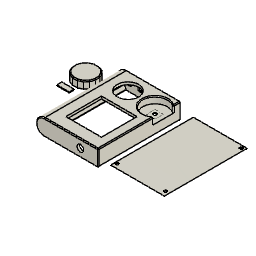
Luxer_main v10 (Autodesk Fusion 360 design; units mm, degrees)
Autodesk Fusion 360 part; units mm, degrees
sketch "草图1" plane through (0, 0, 0) normal (0, 0, 1) x (1, 0, 0)
  line L0 (-40.0171, 49.9772) -> (34.9829, 49.9772)
  line L1 (34.9829, 49.9772) -> (34.9829, -50.0228)
  line L2 (34.9829, -50.0228) -> (-40.0171, -50.0228)
  line L3 (-40.0171, -50.0228) -> (-40.0171, 49.9772)
  circle A0 centre (-8, 29) radius 13
  line L4 (-18.3671, 7.3548) -> (24.6329, 7.3548)
  line L5 (24.6329, 7.3548) -> (24.6329, -35.6452)
  line L6 (24.6329, -35.6452) -> (-18.3671, -35.6452)
  line L7 (-18.3671, -35.6452) -> (-18.3671, 7.3548)
  line L8 (33.5, 48.5) -> (-30, 48.5)
  line L9 (-30, 48.5) -> (-30, -47)
  line L10 (-30, -47) -> (33.5, -47)
  arc A1 (34.9829, 39.8827) -> (34.9829, 18.1173) centre (24.6597, 29) ccw
  arc A2 (34.9829, 41.8647) -> (34.9829, 16.1353) centre (24.6597, 29) ccw
  line L11 (33.5, -47) -> (33.5, 15.0746)
  line L12 (33.5, 42.9254) -> (33.5, 48.5)
  line L13 (33.5, 42.9254) -> (33.5, 15.0746)
  circle A3 centre (24.6597, 29) radius 2
  line L14 (29.7597, 23.9) -> (19.5597, 23.9)
  line L15 (19.5597, 23.9) -> (19.5597, 34.1)
  line L16 (19.5597, 34.1) -> (29.7597, 34.1)
  line L17 (29.7597, 34.1) -> (29.7597, 23.9)
  line L18 (29.7597, 23.9) -> (19.5597, 34.1) construction
  line L19 (19.5597, 23.9) -> (29.7597, 34.1) construction
  circle A4 centre (31.5, 46.5) radius 1.85
  arc A5 (29.5, 48.5) -> (29.4957, 44.7696) centre (30.7332, 46.6334) ccw
  circle A6 centre (30.6894, -44.1882) radius 1.85
  circle A7 centre (-27.5, -44.5) radius 1.85
  arc A8 (-23.5, -47) -> (-30, -40.5) centre (-30, -47) ccw
  arc A9 (33.5, -40) -> (26.5, -47) centre (33.5, -47) ccw
  line L20 (-30, -47) -> (-30, -50.0228)
  line L21 (-30, 48.5) -> (-30, 49.9772)
  point P0 (24.6597, 29)
  dimension "d2" = 75
  dimension "d3" = 100
  dimension "d4" = 26
  dimension "d5" = 15
  dimension "d6" = 43
  dimension "d7" = 43
  dimension "d32" = 4
  dimension "d33" = 10.2
  dimension "d34" = 10.2
  dimension "d63" = 3.7
  dimension "d65" = 3.7
  dimension "d66" = 3.7
  constraint horizontal L0
  constraint vertical L1
  constraint horizontal L2
  constraint vertical L3
  constraint horizontal L4
  constraint vertical L5
  constraint horizontal L6
  constraint vertical L7
  constraint horizontal A0.centre P0
  constraint horizontal L8
  constraint vertical L9
  constraint horizontal L10
  constraint vertical L11
  constraint concentric A1 A2
  constraint coincident L1 A1.end
  constraint coincident L1 A1.start
  constraint coincident L1 A2.end
  constraint coincident L1 A2.start
  constraint coincident A2 L12.start
  constraint collinear L11 L12
  constraint coincident A2 L11.end
  constraint concentric A2 A3
  constraint perpendicular L14 L15
  constraint parallel L14 L16
  constraint parallel L15 L17
  constraint horizontal L14
  constraint coincident L18 P0
  constraint coincident L19 P0
  constraint coincident P0 A1.centre
  constraint coincident L8 A5.start
  constraint coincident A2 A5.end
  constraint coincident L10 A8.start
  constraint coincident L9.end L10.start
  constraint coincident L9 A8.end
  constraint coincident L10 A9.end
  constraint coincident L10.end L11.start
  constraint coincident L11 A9.start
  constraint coincident L2 L20.end
  constraint perpendicular L2 L20
  constraint coincident L0 L21.end
  constraint perpendicular L0 L21
  measures "d2" distance of L0.start L0.end
  measures "d3" distance of L0.start L2.end
  measures "d4" diameter of A0
  measures "d5" radius of A1
  measures "d6" distance of L4.start L4.end
  measures "d7" distance of L4.start L6.end
  measures "d32" diameter of A3
  measures "d33" distance of L15.end L16.end
  measures "d34" distance of L14.end L15.end
  measures "d63" diameter of A4
  measures "d65" diameter of A6
  measures "d66" diameter of A7
extrude "拉伸4" add sketch "草图1" along normal mid plane 20 contours L0 L2 L3 L9 L20 L21 | L0 L1 L8 A2 L12 L21 | L8 L9 L10 A2 L11 A5 A8 A9 | L1 L2 L10 A2 L11 L20 | L1 A1 A2 L13 | L8 A2 L12 A5 | L9 L10 A8 | L1 A1 L13 | A1 A2 L13 | L1 A1 A2 L13 | A1 L13 | L10 L11 A9 | A0 | L4 L5 L6 L7 | A3 | L14 L15 L16 L17 | A4 | A6 | A7 makes body 1
extrude "拉伸5" cut sketch "草图1" along normal blind 17 from surface at -10 contours L8 L9 L10 A2 L11 A5 A8 A9 | L8 A2 L12 A5 | L9 L10 A8 | L10 L11 A9 | A4 | A6 | A7 bodies 1
extrude "拉伸6" add sketch "草图1" along normal blind 17 from surface at -10 contours L8 L9 L10 A2 L11 A5 A8 A9 | L8 A2 L12 A5 | L9 L10 A8 | L10 L11 A9 | A4 | A6 | A7 bodies 1
extrude "拉伸7" cut sketch "草图1" along normal blind 17 from surface at -10 contours L8 L9 L10 A2 L11 A5 A8 A9 | L8 A2 L12 A5 | L9 L10 A8 | L10 L11 A9 | A4 | A6 | A7 bodies 1
extrude "拉伸8" cut sketch "草图1" against normal blind 20 from surface at 10 contours L4 L5 L6 L7 bodies 1
extrude "拉伸9" cut sketch "草图1" against normal blind 20 from surface at 10 contours A0 bodies 1
extrude "拉伸10" cut sketch "草图1" against normal blind 8 from surface at 10 contours L1 A1 L13 | A1 L13 | A3 | L14 L15 L16 L17 bodies 1
extrude "拉伸11" cut sketch "草图1" along normal blind 8 from surface at -10 contours A1 A2 L13 | A1 L13 | A3 | L14 L15 L16 L17 bodies 1
extrude "拉伸12" cut sketch "草图1" along normal blind 3 from surface at -2 contours A3 | L14 L15 L16 L17 bodies 1
extrude "拉伸13" cut sketch "草图1" along normal blind 5 contours A3 bodies 1
fillet "圆角1" radius 10 1 edges at (-40.0171, -0.0228, 10) on bodies 1
fillet "圆角2" radius 10 1 edges at (-40.0171, -0.0228, -10) on bodies 1
fillet "圆角3" radius 1.5 1 edges at (34.9829, -0.0228, -10) on bodies 1
sketch "草图2" plane through (0, 0, 0) normal (0, 1, 0) x (1, 0, 0)
  circle A0 centre (13.5508, -0.0658) radius 4
  circle A1 centre (-26, 0) radius 3.75
  line L0 (4.004, -3.3409) -> (-15.196, -3.3409)
  line L1 (-15.196, -3.3409) -> (-15.196, 3.4591)
  line L2 (-15.196, 3.4591) -> (4.004, 3.4591)
  line L3 (4.004, 3.4591) -> (4.004, -3.3409)
  line L4 (4.004, -3.3409) -> (-15.196, 3.4591) construction
  line L5 (-15.196, -3.3409) -> (4.004, 3.4591) construction
  point P0 (-5.596, 0.0591)
  dimension "d50" = 8
  dimension "d51" = 7.5
  dimension "d84" = 19.2
  dimension "d85" = 6.8
  constraint perpendicular L0 L1
  constraint parallel L0 L2
  constraint parallel L1 L3
  constraint horizontal L0
  constraint coincident L4 P0
  constraint coincident L5 P0
  measures "d50" diameter of A0
  measures "d51" diameter of A1
  measures "d84" distance of L1.end L2.end
  measures "d85" distance of L0.end L1.end
extrude "拉伸23" add sketch "草图1" against normal blind 17 from surface at 7 contours L10 L11 A9 bodies 1
extrude "拉伸24" add sketch "草图1" against normal blind 17 from surface at 7 contours L9 L10 A8 bodies 1
extrude "拉伸25" add sketch "草图1" against normal blind 17 from surface at 7 contours L8 A2 L12 A5 bodies 1
extrude "拉伸26" cut sketch "草图2" along normal blind 58 contours L0 L1 L2 L3 bodies 1
extrude "拉伸27" cut sketch "草图2" along normal blind 57 contours A1 bodies 1
extrude "拉伸28" cut sketch "草图2" against normal blind 60 contours A0 bodies 1
extrude "拉伸29" add sketch "草图1" along normal mid plane 1.4 separate body contours L0 L1 L8 A2 L12 L21 | L8 L9 L10 A2 L11 A5 A8 A9 | L1 L2 L10 A2 L11 L20 | L1 A1 A2 L13 | L8 A2 L12 A5 | L9 L10 A8 | L1 A1 L13 | A1 A2 L13 | L1 A1 A2 L13 | A1 L13 | L10 L11 A9 | A0 | L4 L5 L6 L7 makes body 2
move_body "移动1" bodies 2 to x (1, 0, 0) y (0, 1, 0) z (0, 0, 1) at (80, 0, 0)
delete_face "删除面4" 1 faces at (106.3597, 34.1, -0.2333) on bodies 2
chamfer "倒角1" distance 0.3 angle 45 1 edges at (109.7752, 45.831, -0.7) on bodies 2
chamfer "倒角2" distance 0.3 angle 45 1 edges at (108.9646, -44.8572, -0.7) on bodies 2
chamfer "倒角3" distance 0.3 angle 45 1 edges at (50.7752, -45.169, -0.7) on bodies 2
sketch "草图3" plane through (0, 0, 0) normal (0, 0, 1) x (1, 0, 0)
  line L0 (-51.8552, 41.0396) -> (-57.0064, 42.8573)
  line L1 (-57.0064, 42.8573) -> (-62.4611, 42.5654)
  line L2 (-62.4611, 42.5654) -> (-67.3889, 40.2083)
  line L3 (-67.3889, 40.2083) -> (-71.0396, 36.1448)
  line L4 (-71.0396, 36.1448) -> (-72.8573, 30.9936)
  line L5 (-72.8573, 30.9936) -> (-72.5654, 25.5389)
  line L6 (-72.5654, 25.5389) -> (-70.2083, 20.6111)
  line L7 (-70.2083, 20.6111) -> (-66.1448, 16.9604)
  line L8 (-66.1448, 16.9604) -> (-60.9936, 15.1427)
  line L9 (-60.9936, 15.1427) -> (-55.5389, 15.4346)
  line L10 (-55.5389, 15.4346) -> (-50.6111, 17.7917)
  line L11 (-50.6111, 17.7917) -> (-46.9604, 21.8552)
  line L12 (-46.9604, 21.8552) -> (-45.1427, 27.0064)
  line L13 (-45.1427, 27.0064) -> (-45.4346, 32.4611)
  line L14 (-45.4346, 32.4611) -> (-47.7917, 37.3889)
  line L15 (-47.7917, 37.3889) -> (-51.8552, 41.0396)
  circle A0 centre (-59, 29) radius 1.95
  circle A1 centre (-59, 29) radius 11
  circle A2 centre (-59, 29) radius 5
  line L16 (-66.6051, 1.6351) -> (-51.6051, 1.6351)
  line L17 (-51.6051, 1.6351) -> (-51.6051, 7.6351)
  line L18 (-51.6051, 7.6351) -> (-66.6051, 7.6351)
  line L19 (-66.6051, 7.6351) -> (-66.6051, 1.6351)
  point P0 (-59, 29)
  dimension "d108" = 14
  dimension "d109" = 3.9
  dimension "d125" = 13.8573
  dimension "d126" = 15
  dimension "d127" = 6
  dimension "d128" = 10
  constraint coincident P0 A0.centre
  constraint horizontal L16
  constraint vertical L17
  constraint horizontal L18
  constraint vertical L19
  measures "d108" distance of L0.start P0
  measures "d109" diameter of A0
  measures "d125" horizontal distance of L4.end P0
  measures "d126" distance of L17.end L18.end
  measures "d127" distance of L16.start L18.end
  measures "d128" diameter of A2
extrude "拉伸30" add sketch "草图3" along normal mid plane 9 separate body contours L0 L1 L2 L3 L4 L5 L6 L7 L8 L9 L10 L11 L12 L13 L14 L15 | A0 | A1 | A2 makes body 3
extrude "拉伸31" cut sketch "草图3" along normal blind 7.5 from surface at -4.5 contours A0 bodies 3
extrude "拉伸32" cut sketch "草图3" along normal blind 7.5 from surface at -4.5 contours A1 bodies 3
chamfer "倒角4" distance 1 angle 45 16 edges at (-53.075, 16.6131, 4.5) (-48.7857, 19.8235, 4.5) (-46.0515, 24.4308, 4.5) (-45.2886, 29.7338, 4.5) (-46.6131, 34.925, 4.5) (-49.8235, 39.2143, 4.5) (-54.4308, 41.9485, 4.5) (-59.7338, 42.7114, 4.5) (-64.925, 41.3869, 4.5) (-69.2143, 38.1765, 4.5) (-71.9485, 33.5692, 4.5) (-72.7114, 28.2662, 4.5) (-71.3869, 23.075, 4.5) (-68.1765, 18.7857, 4.5) (-63.5692, 16.0515, 4.5) (-58.2662, 15.2886, 4.5) on bodies 3
fillet "圆角4" radius 0.5 16 edges at (-71.9485, 33.5692, -4.5) (-69.2143, 38.1765, -4.5) (-64.925, 41.3869, -4.5) (-59.7338, 42.7114, -4.5) (-54.4308, 41.9485, -4.5) (-72.7114, 28.2662, -4.5) (-71.3869, 23.075, -4.5) (-68.1765, 18.7857, -4.5) (-63.5692, 16.0515, -4.5) (-58.2662, 15.2886, -4.5) (-53.075, 16.6131, -4.5) (-48.7857, 19.8235, -4.5) (-46.0515, 24.4308, -4.5) (-45.2886, 29.7338, -4.5) (-46.6131, 34.925, -4.5) (-49.8235, 39.2143, -4.5) on bodies 3
extrude "拉伸33" cut 1 faces at (-55.0425, 28.6547, -4.5) along direction (0, 0, 1) blind 0.5 on bodies 3 bodies 3
fillet "圆角5" radius 1.5 4 edges at (114.9829, -0.0228, -0.7) (50, -0.0228, -0.7) (82.4914, -50.0228, -0.7) (82.4914, 49.9772, -0.7) on bodies 2
extrude "拉伸34" add sketch "草图3" along normal mid plane 1 separate body contours L16 L17 L18 L19 makes body 4
fillet "圆角6" radius 1 2 edges at (34.9829, 18.1173, 6) (34.9829, 39.8827, 6) on bodies 1
chamfer "倒角5" distance 1 angle 45 15 edges at (34.9829, -17.0129, 10) (34.4397, 16.8865, 10) (9.6597, 29, 10) (34.4397, 41.1135, 10) (34.9829, 45.9901, 10) (2.4829, 49.9772, 10) (-40.0171, 49.9772, 0) (1.7329, 49.9772, -10) (34.5435, 49.9772, -9.5607) (34.9829, 49.9772, 0.75) (34.9829, -50.0228, 0.75) (34.5435, -50.0228, -9.5607) (1.7329, -50.0228, -10) (-40.0171, -50.0228, 0) (2.4829, -50.0228, 10) on bodies 1
cylinder "圆柱体基本要素1" cut diameter 12.5 height 85 placed x (1, 0, 0) y (0, 0, 1) z (0, -1, 0) at (-30, 48.5, 0) bodies 1
fillet "圆角7" radius 1 2 edges at (-30, 6, 6.25) (-30, 4, 7) on bodies 1
fillet "圆角8" radius 4 1 edges at (-30, 6, -6.25) on bodies 1
delete_face "删除面5" 1 faces at (-22.2686, 49.4848, -0.3734) on bodies 1
extrude "拉伸35" cut sketch "草图2" along normal blind 73 contours A1 bodies 1
fillet "圆角9" radius 2 1 edges at (-29.9683, 6, 6.2499) on bodies 1
extrude "拉伸14" [suppressed]
extrude "拉伸15" [suppressed]
extrude "拉伸16" [suppressed]
extrude "拉伸17" [suppressed]
extrude "拉伸18" [suppressed]
extrude "拉伸19" [suppressed]
extrude "拉伸20" [suppressed]
extrude "拉伸21" [suppressed]
delete_face "删除面1" [suppressed]
delete_face "删除面2" [suppressed]
extrude "拉伸22" [suppressed]
delete_face "删除面3" [suppressed]
